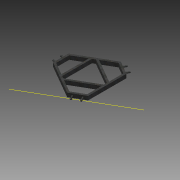
# Autodesk Inventor part: Platform
Saved by Autodesk Inventor 2016 (Build 200138000, 138)
## iProperties
Created: 2016-02-02
Part Number: Platform
Material: Steel
Document SubType Name: Modeling
Designer: tuttlem
Mass: 32237.8 g
Surface Area: 4761.07 cm^2
Volume: 4106.72 cm^3
Density: 7.85 g/cm^3
Appearance: Plate
Author: tuttlem
Autodesk Inventor part; units mm, degrees
ref_plane "YZ Plane" through (0, 0, 0) normal (1, 0, 0) x (0, 1, 0)
ref_plane "XZ Plane" through (0, 0, 0) normal (0, 1, 0) x (-1, 0, 0)
ref_plane "XY Plane" through (0, 0, 0) normal (0, 0, 1) x (1, 0, 0)
sketch "Sketch1" plane through (0, 0, 0) normal (0, 1, 0) x (-1, 0, 0)
  line L0 (613.6799, 122.9576) -> (173.739, 376.9576)
  line L1 (-2.2373, 275.3576) -> (-2.2373, -232.6424)
  line L2 (173.739, -334.2424) -> (613.6799, -80.2424)
  line L3 (613.6799, 122.9576) -> (613.6799, -80.2424)
  line L4 (173.739, 376.9576) -> (-2.2373, 275.3576)
  line L5 (173.739, -334.2424) -> (-2.2373, -232.6424)
  line L6 (588.2799, 108.2929) -> (173.739, 347.6282)
  line L7 (173.739, 347.6282) -> (23.1627, 260.6929)
  line L8 (23.1627, 260.6929) -> (23.1627, -217.9777)
  line L9 (23.1627, -217.9777) -> (173.739, -304.913)
  line L10 (173.739, -304.913) -> (588.2799, -65.5777)
  line L11 (588.2799, -65.5777) -> (588.2799, 108.2929)
  line L12 (397.9021, 218.2076) -> (397.9021, -175.4924)
  line L13 (364.1169, 237.7135) -> (23.1627, 40.8635)
  line L14 (364.1169, -194.9983) -> (23.1627, 1.8517)
  line L15 (338.7169, 252.3782) -> (23.1627, 70.1929)
  line L16 (23.1627, -27.4777) -> (338.7169, -209.663)
  line L17 (423.3021, 203.5429) -> (423.3021, -160.8277)
  point P0 (0, 0)
  dimension "d0" = 203.2
  dimension "d6" = 508
  dimension "d14" = 393.7
  dimension "d16" = 393.7
  dimension "d17" = 393.7
  constraints: 36 end point, 12 point on line, 8 parallel, 6 vertical, 6 other
  measures "d0" distance of L0.start L2.end
  measures "d6" distance of L0.start L0.end
  measures "d14" distance of L12.start L12.end
  measures "d16" distance of L13.start L13.end
  measures "d17" distance of L14.start L14.end
extrude "Extrusion1" add sketch "Sketch1" along normal blind 50.8 contours L3 L2 L5 L1 L4 L0 | L17 L10 L12 L6 | L13 L8 L15 L6 | L10 L16 L8 L14
sketch "Sketch2" plane through (2.2373, 0, 275.3576) normal (0.5, 0, 0.8660254) x (0.8660254, 0, -0.5)
  line L0 (-203.2, 0) -> (0, 0) projected
  line L1 (0, 0) -> (0, 50.8) projected
  line L2 (-203.2, 50.8) -> (0, 50.8) projected
  line L3 (-203.2, 0) -> (-203.2, 50.8) projected
  line L4 (-203.2, 50.8) -> (0, 50.8) projected
  line L5 (-101.6, 50.8) -> (-101.6, 0)
  line L6 (-101.6, 25.4) -> (-152.4, 25.4)
  line L7 (-101.6, 25.4) -> (-50.8, 25.4)
  circle A0 centre (-50.8, 25.4) radius 9.525
  circle A1 centre (-152.4, 25.4) radius 9.525
  point P0 (135.7412, 0)
  dimension "d23" = 50.8
  dimension "d24" = 50.8
  dimension "d25" = 19.05
  dimension "d26" = 19.05
  constraints: 6 end point, 3 midpoint, 2 centre point, 2 coincident, 1 horizontal, 1 point on line
  measures "d23" distance of L6.start L6.end
  measures "d24" distance of L6.start L7.end
  measures "d25" diameter of A0
  measures "d26" diameter of A1
extrude "Extrusion2" add sketch "Sketch2" along normal blind 50.8 contours A0 | A1
sketch "Sketch3" plane through (-173.739, 0, -334.2424) normal (0.5, 0, -0.8660254) x (-0.8660254, 0, -0.5)
  line L0 (-203.2, 0) -> (0, 0) projected
  line L1 (0, 0) -> (0, 50.8) projected
  line L2 (-203.2, 50.8) -> (0, 50.8) projected
  line L3 (-203.2, 0) -> (-203.2, 50.8) projected
  line L4 (152.4, 50.8) -> (-355.6, 50.8) projected
  line L5 (-101.6, 50.8) -> (-101.6, 0)
  line L6 (152.4, 0) -> (-355.6, 0) projected
  line L7 (-101.6, 25.4) -> (-152.4, 25.4)
  line L8 (-101.6, 25.4) -> (-50.8, 25.4)
  circle A0 centre (-50.8, 25.4) radius 9.525
  circle A1 centre (-152.4, 25.4) radius 9.525
  point P0 (-317.5836, 0)
  dimension "d29" = 50.8
  dimension "d30" = 50.8
  dimension "d31" = 19.05
  dimension "d32" = 19.05
  constraints: 6 end point, 3 midpoint, 2 centre point, 2 coincident, 1 horizontal, 1 point on line
  measures "d29" distance of L7.start L7.end
  measures "d30" distance of L7.start L8.end
  measures "d31" diameter of A0
  measures "d32" diameter of A1
extrude "Extrusion3" add sketch "Sketch3" along normal blind 50.8 contours A0 | A1
sketch "Sketch4" plane through (-613.6799, 0, -80.2424) normal (-1, 0, 0) x (0, 0, 1)
  line L0 (150.4353, 0) -> (150.4353, 50.8) projected
  line L1 (0, 0) -> (203.2, 0) projected
  line L2 (203.2, 0) -> (203.2, 50.8) projected
  line L3 (0, 50.8) -> (203.2, 50.8) projected
  line L4 (0, 0) -> (0, 50.8) projected
  line L5 (355.6, 50.8) -> (-152.4, 50.8) projected
  line L6 (101.6, 50.8) -> (101.6, 0)
  line L7 (355.6, 0) -> (-152.4, 0) projected
  line L8 (101.6, 25.4) -> (50.8, 25.4)
  line L9 (101.6, 25.4) -> (152.4, 25.4)
  circle A0 centre (152.4, 25.4) radius 9.525
  circle A1 centre (50.8, 25.4) radius 9.525
  point P0 (80.2424, 0)
  dimension "d35" = 50.8
  dimension "d36" = 50.8
  dimension "d37" = 19.05
  dimension "d38" = 19.05
  constraints: 6 end point, 3 midpoint, 2 centre point, 2 coincident, 1 horizontal, 1 point on line
  measures "d35" distance of L8.start L8.end
  measures "d36" distance of L8.start L9.end
  measures "d37" diameter of A0
  measures "d38" diameter of A1
extrude "Extrusion4" add sketch "Sketch4" along normal blind 50.8 contours A0 L9 L0 | L0 A0 | L9 A0 L0 | A1
sketch "Sketch5" plane through (-16.3568, 25.4, 344.7517) normal (0.5, 0, 0.8660254) x (0.8660254, 0, -0.5)
  circle A0 centre (-101.6, 0) radius 9.525 projected
  circle A1 centre (0, 0) radius 9.525 projected
  arc A2 (-12.7, 0) -> (12.7, 0) centre (0, 0) ccw
  arc A3 (-114.3, 0) -> (-88.9, 0) centre (-101.6, 0) ccw
  line L0 (12.7, 0) -> (-12.7, 0)
  line L1 (-88.9, 0) -> (-114.3, 0)
  point P0 (186.5412, -25.4)
  constraints: 4 end point, 4 point on circle, 2 centre point, 1 collinear, 1 horizontal
revolve "Revolution1" add sketch "Sketch5" angle 360 about axis through (-5.3582, 25.4, 338.4017) along (-0.8660254, 0, 0.5) picked at (-103.4959, -3.3728) picked at (-1.8036, -2.613) contours L1 A3 A0 | A0 L1 | L0 A2 A1 | A1 L0
sketch "Sketch6" plane through (-664.4799, 25.4, 72.1576) normal (-1, 0, 0) x (0, 0, 1)
  circle A0 centre (0, 0) radius 9.525 projected
  circle A1 centre (-101.6, 0) radius 9.525 projected
  arc A2 (-12.7, 0) -> (12.7, 0) centre (0, 0) ccw
  arc A3 (-114.3, 0) -> (-88.9, 0) centre (-101.6, 0) ccw
  line L0 (12.7, 0) -> (-12.7, 0)
  line L1 (-88.9, 0) -> (-114.3, 0)
  point P0 (-72.1576, -25.4)
  constraints: 4 end point, 4 point on circle, 2 centre point, 1 collinear, 1 horizontal
revolve "Revolution2" add sketch "Sketch6" angle 360 about axis through (-664.4799, 25.4, 84.8576) along (0, 0, -1) picked at (-1.8036, -2.613) picked at (-103.4959, -3.3728) contours L0 A2 A0 | A0 L0 | L1 A3 A1 | A1 L1
sketch "Sketch7" plane through (-104.3449, 25.4, -352.8365) normal (0.5, 0, -0.8660254) x (-0.8660254, 0, -0.5)
  circle A0 centre (0, 0) radius 9.525 projected
  circle A1 centre (-101.6, 0) radius 9.525 projected
  arc A2 (-12.7, 0) -> (12.7, 0) centre (0, 0) ccw
  arc A3 (-114.3, 0) -> (-88.9, 0) centre (-101.6, 0) ccw
  line L0 (12.7, 0) -> (-12.7, 0)
  line L1 (-88.9, 0) -> (-114.3, 0)
  point P0 (-266.7836, -25.4)
  constraints: 4 end point, 4 point on circle, 2 centre point, 1 collinear, 1 horizontal
revolve "Revolution3" add sketch "Sketch7" angle 360 about axis through (-115.3435, 25.4, -359.1865) along (0.8660254, 0, 0.5) picked at (-1.8036, -2.613) picked at (-103.4959, -3.3728) contours L0 A2 A0 | A0 L0 | L1 A3 A1 | A1 L1
body "Solid1"
